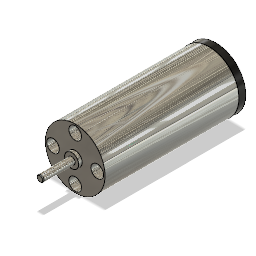
8520 Coreless Motor v3 (Autodesk Fusion 360 design; units mm, degrees)
Autodesk Fusion 360 part; units mm, degrees
sketch "Sketch1" plane through (0, 0, 0) normal (0, 0, 1) x (1, 0, 0)
  circle A0 centre (0, 0) radius 4.25
  dimension "d1" = 8.5
  measures "d1" diameter of A0
extrude "Extrude1" add sketch "Sketch1" along normal blind 20 makes body 1
sketch "Sketch2" plane through (0, 0, 20) normal (0, 0, 1) x (1, 0, 0)
  circle A0 centre (0, 0) radius 4.25
  circle A1 centre (0, 0) radius 0.5
  dimension "d4" = 1
  measures "d4" diameter of A1
extrude "Extrude2" add sketch "Sketch2" along normal blind 5 contours A1 bodies 1
fillet "Fillet2" radius 0.1 1 edges at (-0.4662, -0.1808, 25) on bodies 1
extrude "Extrude3" cut 1 faces at (1.2134, 0.1971, 0) along direction (0, 0, 1) blind 1 on bodies 1 bodies 1
sketch "Sketch3" plane through (0, 0, 1) normal (0, 0, -1) x (-1, 0, 0)
  circle A0 centre (0, 0) radius 4.25
extrude "Extrude4" add sketch "Sketch3" along normal blind 1 separate body makes body 2
sketch "Sketch4" plane through (0, 0, 20) normal (0, 0, 1) x (1, 0, 0)
  circle A0 centre (0, 0) radius 0.5
  circle A1 centre (0, 0) radius 4.25
  circle A2 centre (0, 0) radius 1
  dimension "d13" = 2
  measures "d13" diameter of A2
extrude "Extrude5" add sketch "Sketch4" along normal blind 0.5 contours A2 bodies 1
sketch "Sketch5" plane through (0, 0, 20) normal (0, 0, 1) x (1, 0, 0)
  circle A0 centre (0, 0) radius 1
  circle A1 centre (0, 0) radius 4.25
  circle A2 centre (0.001, -3.1381) radius 0.9
  line L0 (0, 0) -> (0, 0.0971)
  line L1 (0, 0.0971) -> (0, 1.4335) construction
  circle A3 centre (3.1381, 0.001) radius 0.9
  circle A4 centre (-0.001, 3.1381) radius 0.9
  circle A5 centre (-3.1381, -0.001) radius 0.9
  dimension "d16" = 1.8
  dimension "d18" = 360
  measures "d16" diameter of A2
extrude "Extrude6" cut sketch "Sketch5" against normal blind 10 contours A2 | A3 | A4 | A5 bodies 1
